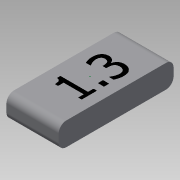
# Autodesk Inventor part: Baterai 1.3
Saved by Autodesk Inventor 2015 SP1 (Build 190203100, 203)
## iProperties
Created: 2015-03-25
Part Number: Baterai 1.3
Material: Generic
Document SubType Name: Modeling
Designer: Rafi Kurnia Putra
Density: 1 g/cm^3
Appearance: Default
Author: Rafi Kurnia Putra
Autodesk Inventor part; units mm, degrees
ref_plane "YZ Plane" through (0, 0, 0) normal (1, 0, 0) x (0, 1, 0)
ref_plane "XZ Plane" through (0, 0, 0) normal (0, 1, 0) x (-1, 0, 0)
ref_plane "XY Plane" through (0, 0, 0) normal (0, 0, 1) x (1, 0, 0)
sketch "Sketch1" plane through (0, 0, 0) normal (0, 0, 1) x (1, 0, 0)
  line L0 (-17, -37.415) -> (17, -37.415)
  line L1 (17, -37.415) -> (17, 37.415)
  line L2 (17, 37.415) -> (-17, 37.415)
  line L3 (-17, 37.415) -> (-17, -37.415)
  line L4 (-17, -37.415) -> (17, 37.415) construction
  line L5 (17, -37.415) -> (-17, 37.415) construction
  point P0 (0, 0)
  dimension "d0" = 34
  dimension "d1" = 74.83
  constraints: 12 end point, 2 midpoint, 2 parallel, 1 horizontal, 1 perpendicular
  measures "d0" distance of L2.end L1.end
  measures "d1" distance of L1.end L0.end
extrude "Extrusion1" add sketch "Sketch1" along normal mid plane 15.09
fillet "Fillet1" radius 5 4 edges at (0, 37.415, -7.545) (0, 37.415, 7.545) (0, -37.415, -7.545) (0, -37.415, 7.545)
sketch "Sketch2" plane through (0, 0, 7.545) normal (0, 0, 1) x (1, 0, 0)
  line L0 (-10.2962, -18.5817) -> (-10.2962, 19.7652) construction
  line L1 (-10.2962, 19.7652) -> (10.5466, 19.7652) construction
  line L2 (10.5466, 19.7652) -> (10.5466, -18.5817) construction
  line L3 (10.5466, -18.5817) -> (-10.2962, -18.5817) construction
  point P0 (0, 0)
  constraints: 2 other
body "Solid1"
